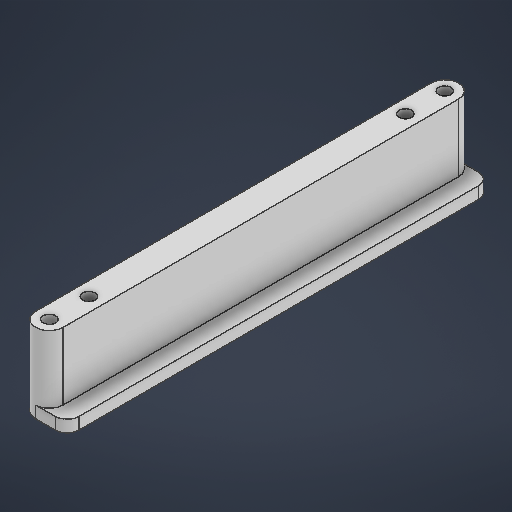
# Autodesk Inventor part: cover_wall_1
Saved by Autodesk Inventor 2026.1 (Build 301233000, 233)
## iProperties
Created: 2026-03-31
Part Number: cover_wall_1
Material: Generic
Document SubType Name: Modeling
Designer: emanuel
Density: 1 g/cm^3
Appearance: Default
Author: emanuel
Autodesk Inventor part; units mm, degrees
ref_plane "YZ Plane" through (0, 0, 0) normal (1, 0, 0) x (0, 1, 0)
ref_plane "XZ Plane" through (0, 0, 0) normal (0, 1, 0) x (-1, 0, 0)
ref_plane "XY Plane" through (0, 0, 0) normal (0, 0, 1) x (1, 0, 0)
sketch "Sketch1" plane through (0, 0, 0) normal (0, 1, 0) x (-1, 0, 0)
  circle A0 centre (0, 0) radius 1.6
  line L0 (0, 0) -> (0, -10)
  circle A1 centre (0, -10) radius 1.6
  line L1 (0, 0) -> (0, 80)
  circle A2 centre (0, 80) radius 1.6
  line L2 (0, 80) -> (0, 90)
  circle A3 centre (0, 90) radius 1.6
  line L3 (0, 90) -> (0, -10) construction
  line L4 (-3.5, 90) -> (-3.5, -10)
  line L5 (3.5, -10) -> (3.5, 90)
  arc A4 (3.5, 90) -> (-3.5, 90) centre (0, 90) ccw
  arc A5 (-3.5, -10) -> (3.5, -10) centre (0, -10) ccw
  point P0 (0, 40)
  dimension "d0" = 3.2
  dimension "d1" = 10
  dimension "d2" = 3.2
  dimension "d3" = 80
  dimension "d4" = 3.2
  dimension "d5" = 10
  dimension "d6" = 3.2
  dimension "d7" = 7
  constraints: 14 end point, 6 centre point, 4 coincident, 4 point on circle, 4 tangent, 4 vertical, 1 midpoint, 1 parallel
  measures "d0" diameter of A0
  measures "d1" distance of L0.start L0.end
  measures "d2" diameter of A1
  measures "d3" distance of L0.start L1.end
  measures "d4" diameter of A2
  measures "d5" distance of L2.start L2.end
  measures "d6" diameter of A3
  measures "d7" diameter of A5
extrude "Extrusion1" add sketch "Sketch1" along normal blind 20
sketch "Sketch2" plane through (0, 0, 0) normal (0, -1, 0) x (1, 0, 0)
  arc A0 (3.5, 90) -> (-3.5, 90) centre (0, 90) ccw projected
  line L0 (0, 93.5) -> (8, 93.5)
  line L1 (8, 93.5) -> (8, -13.5)
  line L2 (8, -13.5) -> (0, -13.5)
  line L3 (0, -13.5) -> (0, 93.5)
  circle A1 centre (0, 90) radius 1.6
  circle A2 centre (0, 80) radius 1.6 projected
  circle A3 centre (0, 80) radius 1.6
  circle A4 centre (0, 0) radius 1.6
  circle A5 centre (0, -9.9761) radius 1.8016
  point P0 (0, 91.6)
  point P1 (0, 88.4)
  point P2 (0, 81.6)
  point P3 (0, 78.4)
  point P4 (0, 1.6)
  point P5 (0, -1.6)
  point P6 (0, -8.1745)
  point P7 (0, -11.7777)
  dimension "d10" = 8
  dimension "d11" = 107
  constraints: 8 end point, 4 centre point, 3 coincident, 2 parallel, 1 horizontal, 1 perpendicular, 1 point on circle, 1 point on line
  measures "d10" distance of L1.end L2.end
  measures "d11" distance of L0.end L1.end
extrude "Extrusion2" add sketch "Sketch2" against normal blind 3 contours L0 L1 L2 L3 A5 A4 A2 A1
fillet "Fillet1" radius 3 2 edges at (8, 1.5, 93.5) (8, 1.5, -13.5)
body "Solid1"
